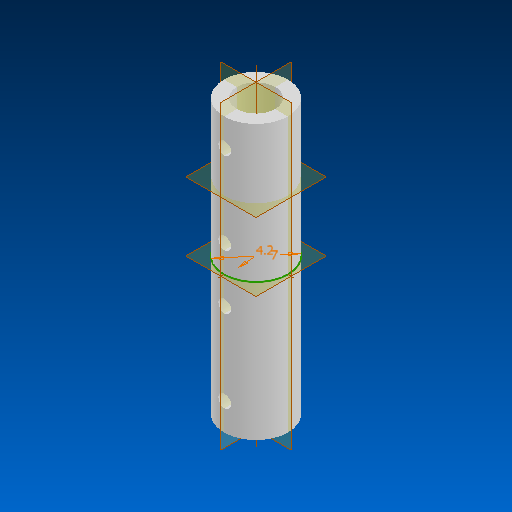
# Autodesk Inventor part: Colletto 3mm
Saved by Autodesk Inventor 2025 (Build 290162000, 162)
## iProperties
Created: 2024-07-23
Part Number: Colletto 3mm
Material: Generic
Document SubType Name: Modeling
Designer: Fabio Ricci
Mass: 0.730287 g
Surface Area: 11.1737 cm^2
Volume: 0.730287 cm^3
Density: 1 g/cm^3
Appearance: Default
Author: Fabio Ricci
## iProperties of the stored document Colletto 3mm_3DPrint.ipt
Created: 2024-07-23
Part Number: Colletto 3mm_3DPrint
Material: Generic
Document SubType Name: Modeling
Designer: Fabio Ricci
Mass: 0.730287 g
Surface Area: 11.1737 cm^2
Volume: 0.730287 cm^3
Density: 1 g/cm^3
Appearance: Default
Author: Fabio Ricci
Autodesk Inventor part; units mm, degrees
sketch "Sketch1" plane through (0, 0, 0) normal (0, 1, 0) x (-1, 0, 0)
  circle A0 centre (0, 0) radius 2.1
  circle A1 centre (0, 0) radius 3.5
  line L0 (0, -2.1) -> (0, -3.5)
  dimension "d0" = 4.2
  dimension "d1" = 7
  constraints: 2 coincident, 2 end point, 2 vertical alignment, 1 vertical, 4 other
extrude "Extrusion1" add sketch "Sketch1" along normal blind 15
sketch "Sketch2" plane through (0, 0, 0) normal (0, 0, 1) x (1, 0, 0)
  point P0 (0, 0)
  point P1 (0.0001, 11.9963)
hole "Hole1" at (0.0001, 11.9963, 0) direction (0, 0, 1) diameter 1.4 depth 4.8 tip angle 118
ref_plane "Work Plane1" through (0, 7.5, 0) normal (0, 1, 0) x (1, 0, 0)
mirror "Mirror1" about plane through (0, 7.5, 0) normal (0, 1, 0) of "Hole1"
mirror "Mirror2" about plane through (0, 0, 0) normal (0, 1, 0) of "Extrusion1"
mirror "Mirror3" about plane through (0, 0, 0) normal (0, 1, 0) of "Hole1", "Mirror1"
body "Solid1"
